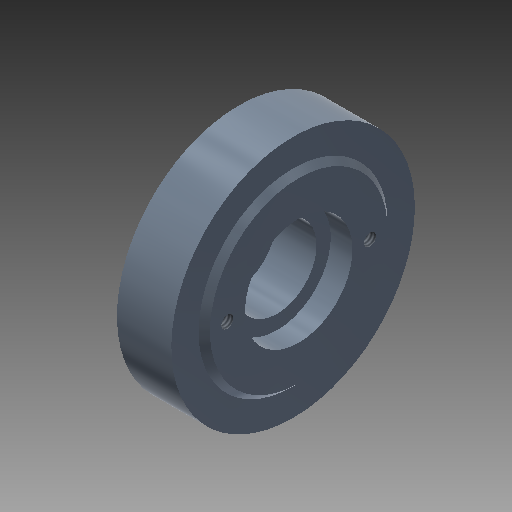
# Autodesk Inventor part: Clutch Housing
Saved by Autodesk Inventor 2017 (Build 210135000, 135)
## iProperties
Created: 2012-08-08
Part Number: Clutch Housing
Material: Stainless Steel, 440C
Document SubType Name: Modeling
Designer: John
Density: 7.75 g/cm^3
Mass: 19.0964 g
Surface Area: 27.3425 cm^2
Volume: 2.46405 cm^3
Appearance: Steel Blue
Author: John
Autodesk Inventor part; units mm, degrees
ref_plane "YZ Plane" through (0, 0, 0) normal (1, 0, 0) x (0, 1, 0)
ref_plane "XZ Plane" through (0, 0, 0) normal (0, 1, 0) x (-1, 0, 0)
ref_plane "XY Plane" through (0, 0, 0) normal (0, 0, 1) x (1, 0, 0)
sketch "Sketch1" plane through (0, 0, 0) normal (1, 0, 0) x (0, 1, 0)
  circle A0 centre (0, 0) radius 14.224
  dimension "d0" = 28.448
  constraints: 1 centre point, 1 coincident
  measures "d0" diameter of A0
extrude "Extrusion1" add sketch "Sketch1" along normal blind 9.9822
sketch "Sketch4" plane through (9.9822, 0, 0) normal (1, 0, 0) x (0, 0, -1)
  circle A0 centre (0, 0) radius 14.224 projected
  circle A1 centre (0, 0) radius 10.3759
  dimension "d10" = 20.7518
  constraints: 1 centre point, 1 coincident
  measures "d10" diameter of A1
extrude "Extrusion4" cut sketch "Sketch4" against normal blind 0.6604
chamfer "Chamfer1" distance 0.6604 angle 45 1 edges at (9.3218, 0, 10.3759)
sketch "Sketch5" plane through (0, 0, 0) normal (-1, 0, 0) x (0, 0, 1)
  circle A0 centre (0, 0) radius 14.224 projected
  circle A1 centre (0, 0) radius 5.461
  dimension "d16" = 10.922
  constraints: 1 centre point, 1 coincident
  measures "d16" diameter of A1
extrude "Extrusion5" cut sketch "Sketch5" against normal blind 2.9718
sketch "Sketch6" plane through (2.9718, 0, 0) normal (-1, 0, 0) x (0, 0, 1)
  circle A0 centre (0, 0) radius 5.461 projected
  circle A1 centre (0, 0) radius 14.224 projected
  circle A2 centre (0, 0) radius 13.0175
  dimension "d19" = 26.035
  constraints: 1 centre point, 1 coincident
  measures "d19" diameter of A2
extrude "Extrusion6" cut sketch "Sketch6" against normal blind 2.5654 contours A2
sketch "Sketch7" plane through (5.5372, 0, 0) normal (-1, 0, 0) x (0, 0, 1)
  circle A0 centre (0, 0) radius 13.0175 projected
  circle A1 centre (0, 0) radius 10.4775
  dimension "d22" = 20.955
  constraints: 1 centre point, 1 coincident
  measures "d22" diameter of A1
extrude "Extrusion7" cut sketch "Sketch7" against normal blind 1.3716
sketch "Sketch8" plane through (0, 0, 0) normal (-1, 0, 0) x (0, 0, 1)
  circle A0 centre (0, 0) radius 5.461 projected
hole "Hole1" at (0, 0, 0) direction (1, 0, 0) diameter 5.08 end through all
sketch "Sketch9" plane through (9.9822, 0, 0) normal (1, 0, 0) x (0, 0, -1)
  circle A0 centre (0, 0) radius 2.54 projected
  circle A1 centre (0, 0) radius 10.3759 projected
  circle A2 centre (0, 0) radius 6.2865
  dimension "d32" = 12.573
  constraints: 1 centre point, 1 coincident
  measures "d32" diameter of A2
extrude "Extrusion8" cut sketch "Sketch9" against normal blind 2.54 contours A2
sketch "Sketch10" plane through (9.9822, 0, 0) normal (1, 0, 0) x (0, 0, -1)
  circle A0 centre (0, 0) radius 10.3759 projected
  circle A1 centre (0, 0) radius 4.6355
  dimension "d35" = 9.271
  constraints: 1 centre point, 1 coincident
  measures "d35" diameter of A1
extrude "Extrusion9" cut sketch "Sketch10" against normal blind 7.3152 contours A1
sketch "Sketch11" plane through (9.9822, 0, 0) normal (1, 0, 0) x (0, 0, -1)
  circle A0 centre (0, 0) radius 6.2865 projected
  circle A1 centre (0, 0) radius 10.3759 projected
  line L0 (0, -10.3759) -> (0, -6.2865)
  line L1 (0, -6.2865) -> (0, 0) construction
  line L2 (0, 6.2865) -> (0, 0) construction
  line L3 (0, 10.3759) -> (0, 6.2865)
  point P0 (0, -8.3312)
  point P1 (0, 8.3312)
  constraints: 8 end point, 5 point on circle, 4 collinear, 2 midpoint, 1 point on line, 1 vertical
hole "Hole2" at (9.9822, -8.3312, 0) at (9.9822, 8.3312, 0) direction (-1, 0, 0) diameter 1.4224 end through all
body "Solid1"
